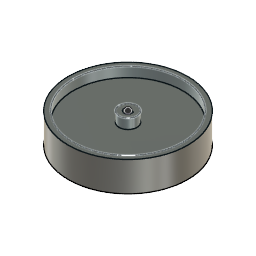
wheel (Autodesk Fusion 360 design; units mm, degrees)
part number: 2026-05-16-09-54-54-859
Autodesk Fusion 360 part; units mm, degrees
sketch "Sketch1" plane through (0, 0, 0) normal (0, 0, 1) x (1, 0, 0)
  circle A0 centre (0, 0) radius 30
  circle A1 centre (0, 0) radius 2
  line L0 (-1.7356, 0.9939) -> (1.7641, 0.9424)
  dimension "d1" = 60
  dimension "d2" = 4
  dimension "d3" = 3.5
  constraint coincident A0.centre A1.centre
  constraint coincident A1 L0.start
  constraint coincident A1 L0.end
  measures "d1" diameter of A0
  measures "d2" diameter of A1
  measures "d3" distance of L0.start L0.end
extrude "Extrude1" add sketch "Sketch1" along normal blind 15 contours A0 | A1 L0 picked at (-0.2335, 1.4513)
sketch "Sketch2" plane through (0, 0, 15) normal (0, 0, 1) x (-1, 0, 0)
  arc A0 (1.7356, -0.9939) -> (-1.7641, -0.9424) centre (0, 0) ccw
  line L0 (1.7356, -0.9939) -> (-1.7641, -0.9424)
  circle A1 centre (0, 0) radius 30
  circle A2 centre (0, 0) radius 4.5
  circle A3 centre (0, 0) radius 27.5
  dimension "d6" = 9
  dimension "d7" = 55
  constraint concentric A0 A2
  constraint coincident A0.centre A1.centre
  measures "d6" diameter of A2
  measures "d7" diameter of A3
extrude "Extrude2" cut sketch "Sketch2" against normal blind 5 contours A3
sketch "Sketch3" plane through (0, 0, 0) normal (0, 0, 1) x (1, 0, 0)
  circle A0 centre (0, 0) radius 4.5
  circle A1 centre (0, 0) radius 27.5
  dimension "d10" = 9
  dimension "d11" = 55
  constraint coincident A0.centre A1.centre
  measures "d10" diameter of A0
  measures "d11" diameter of A1
extrude "Extrude3" cut sketch "Sketch3" along normal blind 5
